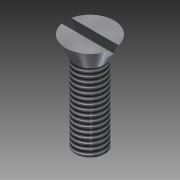
# Autodesk Inventor part: Screw_CountersunkHead_3x10
Saved by Autodesk Inventor 2014 SP1 (Build 180222100, 222)
## iProperties
Created: 2015-03-22
Part Number: Screw_CountersunkHead_3x10
Material: Generic
Document SubType Name: Modeling
Designer: david
Density: 1 g/cm^3
Appearance: Default
Author: david
Autodesk Inventor part; units mm, degrees
ref_plane "YZ Plane" through (0, 0, 0) normal (1, 0, 0) x (0, 1, 0)
ref_plane "XZ Plane" through (0, 0, 0) normal (0, 1, 0) x (-1, 0, 0)
ref_plane "XY Plane" through (0, 0, 0) normal (0, 0, 1) x (1, 0, 0)
sketch "Sketch1" plane through (0, 0, 0) normal (0, 1, 0) x (-1, 0, 0)
  circle A0 centre (0, 0) radius 1.5
  dimension "d0" = 3
  constraints: 1 centre point, 1 coincident
  measures "d0" diameter of A0
extrude "Extrusion1" add sketch "Sketch1" along normal blind 8
thread "Thread1" size "M3x0.5" class "6g" standard "ANSI Metric M Profile" full length
ref_plane "Work Plane1" through (0, 10, 0) normal (0, 1, 0) x (1, 0, 0)
sketch "Sketch4" plane through (0, 10, 0) normal (0, 1, 0) x (1, 0, 0)
  circle A0 centre (0, 0) radius 2.5
  dimension "d14" = 5
  constraints: 1 centre point, 1 coincident
  measures "d14" diameter of A0
loft "Loft1" add profiles "Sketch4" section 2 edges at (1.5, 8, 0)
sketch "Sketch5" plane through (0, 10, 0) normal (0, 1, 0) x (1, 0, 0)
  circle A0 centre (0, 0) radius 2.5 projected
  line L0 (-2.4495, 0.5) -> (2.4495, 0.5)
  line L1 (-2.4495, -0.5) -> (2.4495, -0.5)
  line L2 (0, 0) -> (2.0973, 0) construction
  dimension "d19" = 1
  constraints: 6 end point, 4 point on circle, 2 parallel, 1 horizontal, 1 other
  measures "d19" distance between parallel lines of L1 L0
extrude "Extrusion4" cut sketch "Sketch5" against normal blind 1 contours A0 L1 L0
body "Solid1"
